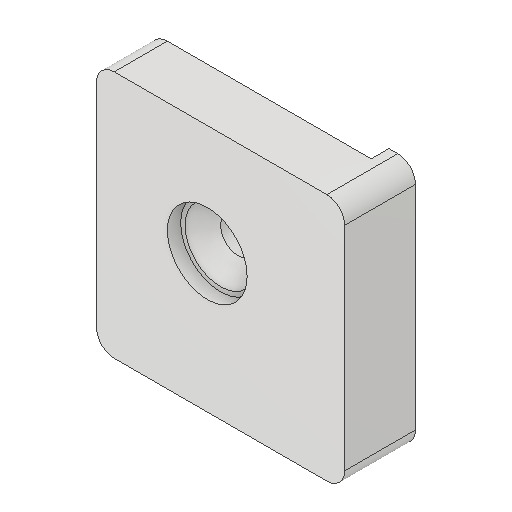
# Autodesk Inventor part: 3DP_PLA_Base_plate_corner_leg
Saved by Autodesk Inventor 2026.1 (Build 301233000, 233)
## iProperties
Created: 2018-07-11
Part Number: 3DP_PLA_Base_plate_corner_leg
Material: ABS Plastic
Document SubType Name: Modeling
Designer: Andrzej
Density: 1.06 g/cm^3
Appearance: Smooth - White
Author: Andrzej
Autodesk Inventor part; units mm, degrees
ref_plane "YZ Plane" through (0, 0, 0) normal (1, 0, 0) x (0, 1, 0)
ref_plane "XZ Plane" through (0, 0, 0) normal (0, 1, 0) x (-1, 0, 0)
ref_plane "XY Plane" through (0, 0, 0) normal (0, 0, 1) x (1, 0, 0)
sketch "Sketch1" plane through (0, 0, 0) normal (0, 0, 1) x (1, 0, 0)
  line L0 (-6.0954, 5.4228) -> (18.9046, 5.4228)
  line L1 (18.9046, 5.4228) -> (18.9046, -19.5772)
  line L2 (18.9046, -19.5772) -> (-6.0954, -19.5772)
  line L3 (-6.0954, -19.5772) -> (-6.0954, 5.4228)
  line L4 (-6.0954, -22.5772) -> (21.9046, -22.5772)
  line L5 (21.9046, -22.5772) -> (21.9046, 5.4228)
  line L6 (18.9046, 5.4228) -> (21.9046, 5.4228)
  line L7 (-6.0954, -19.5772) -> (-6.0954, -22.5772)
  point P0 (0, 0)
  point P1 (6.4046, -7.0772)
  dimension "d0" = 25
  dimension "d1" = 25
  dimension "d2" = 3
  dimension "d3" = 3
  dimension "d4" = 12.5
  dimension "d5" = 12.5
  constraints: 16 end point, 3 perpendicular, 2 parallel, 1 horizontal
  measures "d0" distance of L1.end L2.end
  measures "d1" distance of L0.end L1.end
  measures "d2" distance between parallel lines of L2 L4
  measures "d3" distance between parallel lines of L5 L1
  measures "d4" distance from line of L3 point (6.405, -7.077)
  measures "d5" distance from line of L0 point (6.405, -7.077)
extrude "Extrusion1" add sketch "Sketch1" along normal blind 6
extrude "Extrusion2" add sketch "Sketch1" against normal blind 2 contours L6 L5 L4 L7 L2 L1
hole "Hole1" at (6.4046, -7.0772, 0) direction (0, 0, 1) diameter 4 end through all
sketch "Sketch2" plane through (0, 0, 6) normal (0, 0, 1) x (1, 0, 0)
  circle A0 centre (6.4046, -7.0772) radius 2 projected
  line L0 (-6.0954, 5.4228) -> (-6.0954, -22.5772) projected
  line L1 (-6.0954, -22.5772) -> (21.9046, -22.5772) projected
  line L2 (21.9046, -22.5772) -> (21.9046, 5.4228) projected
  line L3 (21.9046, 5.4228) -> (-6.0954, 5.4228) projected
  circle A1 centre (6.4046, -7.0772) radius 2 projected
  circle A2 centre (6.4046, -7.0772) radius 4.5
  point P0 (0, 0)
  dimension "d17" = 9
  constraints: 1 centre point, 1 coincident
  measures "d17" diameter of A2
extrude "Extrusion3" cut sketch "Sketch2" against normal blind 1.5 contours A2
chamfer "Chamfer1" distance 2 angle 45 1 edges at (6.4046, -9.0772, 4.5)
fillet "Fillet1" radius 2 2 edges at (21.9046, -22.5772, 2) (-6.0954, 5.4228, 3)
equation "\"d4\" = 0.5 * d0"
body "Solid1"
